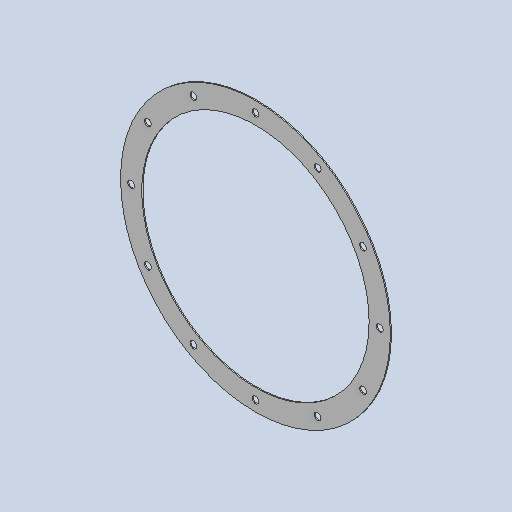
# Autodesk Inventor part: DMF2.0 01 45 Gear ring 5
Saved by Autodesk Inventor 2025 (Build 290162010, 162A)
## iProperties
Created: 2024-04-30
Part Number: DMF2.0 01 45 Gear ring 5
Material: Generic
Document SubType Name: Sheet Metal
Designer: admin
Stock Number: Барабан_Сектор_Усилителя
Density: 1 g/cm^3
Sheet Metal Rule: Default
Sheet Metal Width: 0,000 mm
Sheet Metal Length: 0,000 mm
Sheet Metal Area: 0,000 mm^2
Appearance: Default
Author: pokla
Autodesk Inventor part; units mm, degrees
ref_plane "YZ Plane" through (0, 0, 0) normal (1, 0, 0) x (0, 1, 0)
ref_plane "XZ Plane" through (0, 0, 0) normal (0, 1, 0) x (-1, 0, 0)
ref_plane "XY Plane" through (0, 0, 0) normal (0, 0, 1) x (1, 0, 0)
sketch "Sketch1" plane through (0, 0, 0) normal (0, 0, 1) x (1, 0, 0)
  circle A0 centre (0, 0) radius 214
  circle A1 centre (0, 0) radius 254
  dimension "d31" = 508
  dimension "d32" = 428
  measures "d31" diameter of A1
  measures "d32" diameter of A0
extrude "Plate1" add sketch "Sketch1" against normal blind 2
sketch "Sketch2" plane through (0, 0, 0) normal (0, 0, 1) x (1, 0, 0)
  circle A0 centre (0, 0) radius 214 construction
  circle A1 centre (0, 0) radius 254 construction
  line L0 (0, 254) -> (0, 214) construction
  circle A2 centre (0, 234) radius 6.5
  dimension "d33" = 13
  constraints: 3 vertical alignment, 2 end point, 1 centre point, 1 midpoint, 1 vertical, 2 other
  measures "d33" diameter of A2
extrude "Cut1" cut sketch "Sketch2" against normal blind 2
pattern_circular "Circular Pattern1" count 12 over 360 about axis through (0, 0, 0) along (0, 0, -1) of "Cut1"
equation "\"d31\" = Колесо_диам_3"
equation "\"d32\" = Колесо_диам_4"
equation "\"d34\" = Thickness"
equation "\"d15\" = Thickness"
equation "\"BendRadius\" = Thickness"
equation "\"BendReliefWidth\" = Thickness"
equation "\"BendReliefDepth\" = 0.5 * Thickness"
equation "\"CornerReliefSize\" = 4 * Thickness"
equation "\"MinimumRemnant\" = 2 * Thickness"
equation "\"TransitionRadius\" = BendRadius"
equation "\"JacobiRadiusSize\" = BendRadius"
equation "\"GapSize\" = Thickness"
equation "\"Колесо_диам_3\" = 508"
equation "\"Колесо_диам_4\" = 428"
equation "\"Thickness\" = 2"
body "Solid1"
